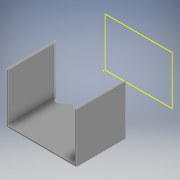
# Autodesk Inventor part: Component box Bottom tall R
Saved by Autodesk Inventor 2021 (Build 250183000, 183)
## iProperties
Created: 2023-01-12
Part Number: Component box Bottom tall R
Material: Generic
Document SubType Name: Modeling
Designer: boyle
Density: 1 g/cm^3
Appearance: Default
Author: boyle
Autodesk Inventor part; units mm, degrees
ref_plane "YZ Plane" through (0, 0, 0) normal (1, 0, 0) x (0, 1, 0)
ref_plane "XZ Plane" through (0, 0, 0) normal (0, 1, 0) x (-1, 0, 0)
ref_plane "XY Plane" through (0, 0, 0) normal (0, 0, 1) x (1, 0, 0)
sketch "Sketch1" plane through (0, 0, 0) normal (0, 1, 0) x (-1, 0, 0)
  line L0 (0, 0) -> (-177.8, 0)
  line L1 (-177.8, 0) -> (-177.8, 254)
  line L2 (-177.8, 254) -> (0, 254)
  line L3 (0, 254) -> (0, 0)
  dimension "d0" = 177.8
  dimension "d1" = 254
  constraints: 8 end point, 2 parallel, 1 horizontal, 1 perpendicular
  measures "d0" distance of L1.end L2.end
  measures "d1" distance of L0.end L1.end
extrude "Extrusion1" add sketch "Sketch1" along normal blind 127
shell "Shell1" thickness 3.81 removed faces 1 at (118.5333, 127, 169.3333)
sketch "Sketch2" plane through (0, 0, 254) normal (0, 0, 1) x (1, 0, 0)
  line L0 (0, 0) -> (177.8, 0) projected
  line L1 (177.8, 0) -> (177.8, 127) projected
  line L2 (0, 127) -> (177.8, 127) projected
  line L3 (0, 0) -> (0, 127) projected
extrude "Extrusion2" cut sketch "Sketch2" against normal up to surface (3.81 mm away)
sketch "Sketch3" plane through (3.81, 3.81, 3.81) normal (0, 0, 1) x (1, 0, 0)
  line L0 (170.18, 0) -> (0, 0) projected
  line L1 (170.18, 0) -> (170.18, 123.19) projected
  line L2 (0, 123.19) -> (170.18, 123.19) projected
  line L3 (0, 0) -> (0, 123.19) projected
  point P0 (-3.81, -3.81)
sketch "Sketch4" plane through (0, 0, 0) normal (0, -1, 0) x (1, 0, 0)
  line L0 (0, 0) -> (0, 250.19) projected
  line L1 (177.8, 0) -> (0, 0) projected
  line L2 (177.8, 250.19) -> (177.8, 0) projected
  line L3 (177.8, 250.19) -> (0, 250.19) projected
  line L4 (0, 0) -> (0, 250.19) projected
  line L5 (177.8, 0) -> (0, 0) projected
  line L6 (177.8, 250.19) -> (177.8, 0) projected
  line L7 (177.8, 250.19) -> (177.8, 0) projected
  spline S0 degree 4 poles (0, 125.095) (18.5625, 164.2011) (32.6327, 79.9754) (47.4518, 162.5292) (113.1446, 101.2486) (116.8423, 161.5015) (155.6163, 85.0462) (160.2364, 161.9134) (177.8, 125.095) knots 0 0 0 0 0 0.323542 0.454905 0.586595 0.711733 1 1 1 1 1
  point P0 (22.8108, 131.2197)
  point P1 (39.2238, 120.7725)
  point P2 (67.4765, 130.2672)
  point P3 (109.2766, 120.6567)
  point P4 (120.9714, 130.8461)
  point P5 (139.1504, 122.7409)
  point P6 (157.2136, 130.7303)
  constraints: 2 midpoint, 9 other
extrude "Extrusion3" cut sketch "Sketch4" against normal through all contours L0 S0 L2 L1
body "Solid1"
